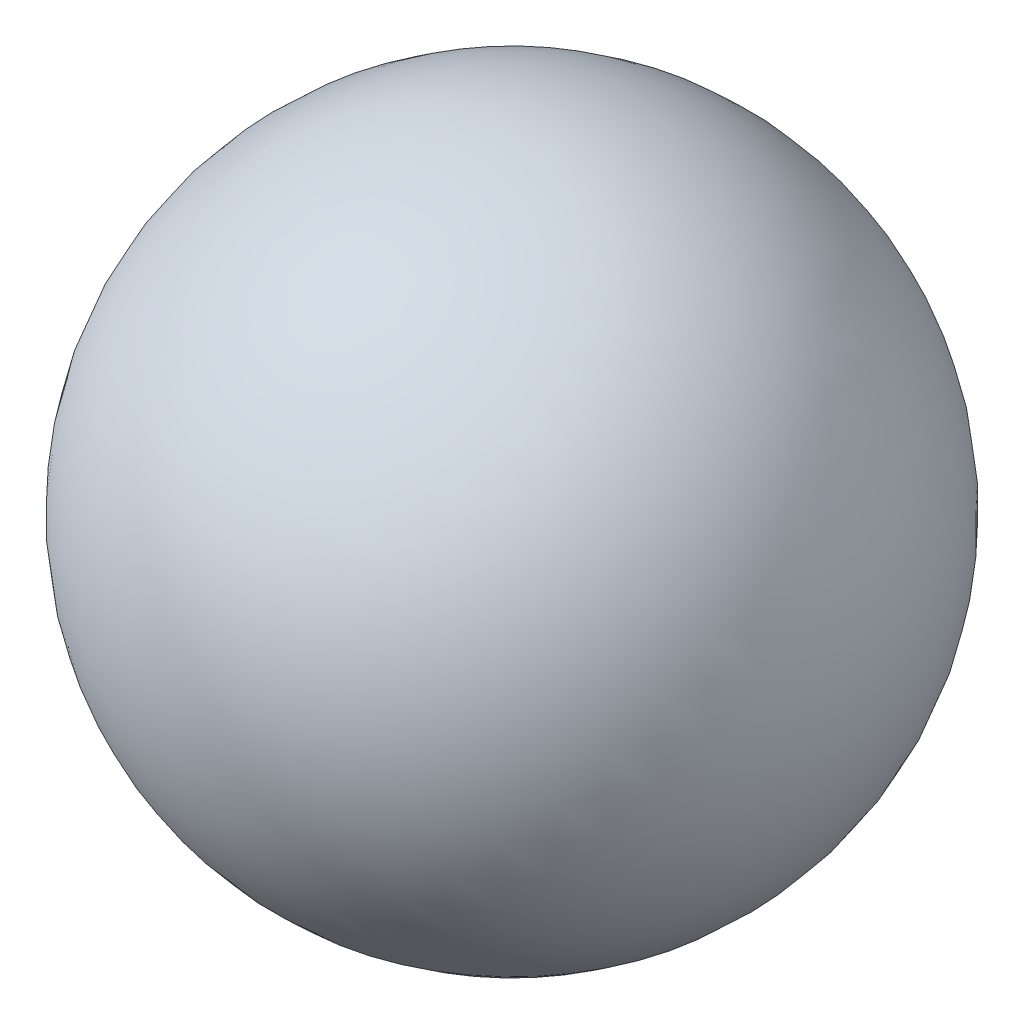
Minge (Autodesk Fusion 360 design; units mm, degrees)
part number: 2026-06-02-22-23-14-859
Autodesk Fusion 360 part; units mm, degrees
sphere "SpherePrimitive1" add diameter 15 placed x (-1, 0, 0) y (0, -1, 0) z (0, 0, 1) at (-33.1301, 120.7399, -10.5153)
